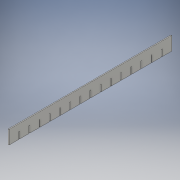
# Autodesk Inventor part: DividerWidthPlastic
Saved by Autodesk Inventor 2016 (Build 200138000, 138)
## iProperties
Created: 2016-02-08
Part Number: DividerWidthPlastic
Material: ABS Plastic
Document SubType Name: Modeling
Designer: ron
Density: 1.06 g/cm^3
Appearance: Smooth - White
Mass: 100.151 g
Surface Area: 661.289 cm^2
Volume: 94.4817 cm^3
Author: ron
Autodesk Inventor part; units mm, degrees
ref_plane "YZ Plane" through (0, 0, 0) normal (1, 0, 0) x (0, 1, 0)
ref_plane "XZ Plane" through (0, 0, 0) normal (0, 1, 0) x (-1, 0, 0)
ref_plane "XY Plane" through (0, 0, 0) normal (0, 0, 1) x (1, 0, 0)
sketch "Sketch1" plane through (0, 0, 0) normal (1, 0, 0) x (0, 1, 0)
  line L0 (0, 0) -> (50.8, 0)
  line L1 (50.8, 0) -> (50.8, -609.6)
  line L2 (50.8, -609.6) -> (0, -609.6)
  line L3 (0, -609.6) -> (0, -573.0875)
  line L4 (0, -573.0875) -> (25.4, -573.0875)
  line L5 (25.4, -573.0875) -> (25.4, -569.9125)
  line L6 (25.4, -569.9125) -> (0, -569.9125)
  line L7 (0, -569.9125) -> (0, -534.9875)
  line L8 (0, -534.9875) -> (25.4, -534.9875)
  line L9 (25.4, -534.9875) -> (25.4, -531.8125)
  line L10 (25.4, -531.8125) -> (0, -531.8125)
  line L11 (0, -531.8125) -> (0, -496.8875)
  line L12 (0, -496.8875) -> (25.4, -496.8875)
  line L13 (25.4, -496.8875) -> (25.4, -493.7125)
  line L14 (25.4, -493.7125) -> (0, -493.7125)
  line L15 (0, -493.7125) -> (0, -458.7875)
  line L16 (0, -458.7875) -> (25.4, -458.7875)
  line L17 (25.4, -458.7875) -> (25.4, -455.6125)
  line L18 (25.4, -455.6125) -> (0, -455.6125)
  line L19 (0, -455.6125) -> (0, -420.6875)
  line L20 (0, -420.6875) -> (25.4, -420.6875)
  line L21 (25.4, -420.6875) -> (25.4, -417.5125)
  line L22 (25.4, -417.5125) -> (0, -417.5125)
  line L23 (0, -417.5125) -> (0, -382.5875)
  line L24 (0, -382.5875) -> (25.4, -382.5875)
  line L25 (25.4, -382.5875) -> (25.4, -379.4125)
  line L26 (25.4, -379.4125) -> (0, -379.4125)
  line L27 (0, -379.4125) -> (0, -344.4875)
  line L28 (0, -344.4875) -> (25.4, -344.4875)
  line L29 (25.4, -344.4875) -> (25.4, -341.3125)
  line L30 (25.4, -341.3125) -> (0, -341.3125)
  line L31 (0, -341.3125) -> (0, -306.3875)
  line L32 (0, -306.3875) -> (25.4, -306.3875)
  line L33 (25.4, -306.3875) -> (25.4, -303.2125)
  line L34 (25.4, -303.2125) -> (0, -303.2125)
  line L35 (0, -303.2125) -> (0, -268.2875)
  line L36 (0, -268.2875) -> (25.4, -268.2875)
  line L37 (25.4, -268.2875) -> (25.4, -265.1125)
  line L38 (25.4, -265.1125) -> (0, -265.1125)
  line L39 (0, -265.1125) -> (0, -230.1875)
  line L40 (0, -230.1875) -> (25.4, -230.1875)
  line L41 (25.4, -230.1875) -> (25.4, -227.0125)
  line L42 (25.4, -227.0125) -> (0, -227.0125)
  line L43 (0, -227.0125) -> (0, -192.0875)
  line L44 (0, -192.0875) -> (25.4, -192.0875)
  line L45 (25.4, -192.0875) -> (25.4, -188.9125)
  line L46 (25.4, -188.9125) -> (0, -188.9125)
  line L47 (0, -188.9125) -> (0, -153.9875)
  line L48 (0, -153.9875) -> (25.4, -153.9875)
  line L49 (25.4, -153.9875) -> (25.4, -150.8125)
  line L50 (25.4, -150.8125) -> (0, -150.8125)
  line L51 (0, -150.8125) -> (0, -115.8875)
  line L52 (0, -115.8875) -> (25.4, -115.8875)
  line L53 (25.4, -115.8875) -> (25.4, -112.7125)
  line L54 (25.4, -112.7125) -> (0, -112.7125)
  line L55 (0, -112.7125) -> (0, -77.7875)
  line L56 (0, -77.7875) -> (25.4, -77.7875)
  line L57 (25.4, -77.7875) -> (25.4, -74.6125)
  line L58 (25.4, -74.6125) -> (0, -74.6125)
  line L59 (0, -74.6125) -> (0, -39.6875)
  line L60 (0, -39.6875) -> (25.4, -39.6875)
  line L61 (25.4, -39.6875) -> (25.4, -36.5125)
  line L62 (25.4, -36.5125) -> (0, -36.5125)
  line L63 (0, -36.5125) -> (0, 0)
  dimension "d293" = 50.8
  dimension "d294" = 609.6
  dimension "d369" = 25.4
  dimension "d371" = 25.4
  dimension "d373" = 25.4
  dimension "d376" = 25.4
  dimension "d378" = 25.4
  dimension "d380" = 25.4
  dimension "d383" = 25.4
  dimension "d385" = 25.4
  dimension "d387" = 25.4
  dimension "d390" = 25.4
  dimension "d392" = 25.4
  dimension "d394" = 25.4
  dimension "d397" = 25.4
  dimension "d399" = 25.4
  dimension "d401" = 25.4
  dimension "d404" = 25.4
  dimension "d406" = 25.4
  dimension "d408" = 25.4
  dimension "d411" = 25.4
  dimension "d413" = 25.4
  dimension "d415" = 25.4
  dimension "d418" = 25.4
  dimension "d420" = 25.4
  constraints: 128 end point, 37 point on line, 25 perpendicular, 8 vertical, 7 parallel, 1 horizontal
  measures "d293" distance of L0.start L0.end
  measures "d294" distance of L0.end L1.end
  measures "d369" distance of L3.end L4.end
  measures "d371" distance of L5.end L6.end
  measures "d373" distance of L7.end L8.end
  measures "d376" distance of L11.end L12.end
  measures "d378" distance of L13.end L14.end
  measures "d380" distance of L15.end L16.end
  measures "d383" distance of L19.end L20.end
  measures "d385" distance of L21.end L22.end
  measures "d387" distance of L23.end L24.end
  measures "d390" distance of L27.end L28.end
  measures "d392" distance of L29.end L30.end
  measures "d394" distance of L31.end L32.end
  measures "d397" distance of L35.end L36.end
  measures "d399" distance of L37.end L38.end
  measures "d401" distance of L39.end L40.end
  measures "d404" distance of L43.end L44.end
  measures "d406" distance of L45.end L46.end
  measures "d408" distance of L47.end L48.end
  measures "d411" distance of L51.end L52.end
  measures "d413" distance of L53.end L54.end
  measures "d415" distance of L55.end L56.end
  measures "d418" distance of L59.end L60.end
  measures "d420" distance of L61.end L62.end
extrude "Extrusion3" add sketch "Sketch1" along normal blind 3.175
body "Solid3"
